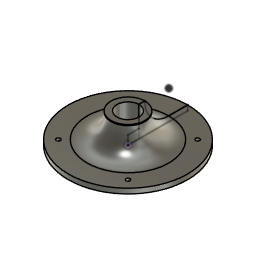
bearing holder (Autodesk Fusion 360 design; units mm, degrees)
Autodesk Fusion 360 part; units mm, degrees
sketch "Sketch1" plane through (0, 0, 0) normal (1, 0, 0) x (0, 1, 0)
  line L0 (0, 0) -> (11, 0) construction
  line L1 (0, 0) -> (60, 0)
  line L2 (60, 0) -> (60, 5)
  line L3 (60, 5) -> (41, 5) construction
  line L4 (0, 5) -> (0, 0) construction
  line L5 (0, 0) -> (0, 9)
  line L6 (11, 0) -> (11, 30) construction
  line L7 (0, 9) -> (11, 9)
  line L8 (11, 9) -> (11, 30)
  line L9 (11, 30) -> (17, 30)
  line L10 (17, 30) -> (17, 29)
  arc A0 (17, 29) -> (41, 5) centre (41, 29) ccw
  line L11 (41, 5) -> (60, 5)
  dimension "d1" = 11
  dimension "d2" = 60
  dimension "d3" = 5
  dimension "d4" = 9
  dimension "d5" = 30
  dimension "d6" = 6
  dimension "d7" = 24
  constraint coincident L0.start L1.start
  constraint horizontal L0
  constraint parallel L0 L1
  constraint perpendicular L1 L2
  constraint perpendicular L2 L3
  constraint perpendicular L1 L4
  constraint perpendicular L3 L5
  constraint perpendicular L1 L6
  constraint coincident L6 L7.end
  constraint perpendicular L6 L7
  constraint perpendicular L6 L9
  constraint perpendicular L3 L10
  constraint coincident L4.start L3
  constraint tangent L10 A0
  constraint tangent L3 A0
  measures "d1" distance of L0.start L0.end
  measures "d2" distance of L0.start L1.end
  measures "d3" distance of L1.end L2.end
  measures "d4" distance of L0.start L5.end
  measures "d5" distance of L0.end L6.end
  measures "d6" distance of L6.end L9.end
  measures "d7" radius of A0
revolve "Revolve1" add sketch "Sketch1" angle 360 about axis through (0, 0, 5) along (0, 0, -1)
sketch "Sketch2" plane through (0, 0, 5) normal (0, 0, 1) x (-1, 0, 0)
  circle A0 centre (0, 0) radius 41
  circle A1 centre (0, 0) radius 60
  line L0 (0, 0) -> (0, 35) construction
  line L1 (0, 0) -> (-35, 0) construction
  line L2 (-35, 0) -> (-35, 35) construction
  line L3 (-35, 35) -> (0, 35) construction
  circle A2 centre (-35, 35) radius 2
  circle A3 centre (-35, -35) radius 2
  circle A4 centre (35, -35) radius 2
  circle A5 centre (35, 35) radius 2
  dimension "d9" = 35
  dimension "d10" = 35
  dimension "d11" = 4
  dimension "d13" = 360
  constraint coincident A0.centre A1.centre
  constraint vertical L0
  constraint perpendicular L0 L1
  constraint perpendicular L1 L2
  constraint perpendicular L0 L3
  constraint coincident L2.end L3.start
  measures "d9" distance of A0.centre L0.end
  measures "d10" distance of A0.centre L1.end
  measures "d11" diameter of A2
extrude "Extrude2" cut sketch "Sketch2" against normal blind 6 contours A2 | A3 | A4 | A5
